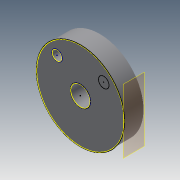
# Autodesk Inventor part: gearSupport
Saved by Autodesk Inventor 2015 (Build 190159000, 159)
## iProperties
Created: 2014-08-31
Part Number: gearSupport
Material: Generic
Document SubType Name: Modeling
Designer: shohei
Density: 1 g/cm^3
Appearance: Default
Author: shohei
Autodesk Inventor part; units mm, degrees
ref_plane "XZ Plane" through (0, 0, 0) normal (0, 1, 0) x (-1, 0, 0)
ref_plane "XY Plane" through (0, 0, 0) normal (0, 0, 1) x (1, 0, 0)
sketch "Block1" plane through (0, 0, 0) normal (0, 0, 1) x (1, 0, 0)
  circle A0 centre (0, 0) radius 20.22
  circle A1 centre (0, 12) radius 2.72
  circle A2 centre (0, 0) radius 5.22
  circle A3 centre (0, -12) radius 2.72
sketch "Block2" plane through (0, 0, 0) normal (0, 0, 1) x (1, 0, 0)
  circle A0 centre (0, 0) radius 22.72
  circle A1 centre (-12, 12) radius 2.72
  circle A2 centre (0, 0) radius 5.22
  point P0 (-4, 4)
sketch "Sketch1" plane through (0, 0, 0) normal (0, 1, 0) x (-1, 0, 0)
  circle A0 centre (0, 0) radius 22.5
  circle A1 centre (0, 0) radius 5
  line L0 (31.5, 0) -> (-31.5, 0) projected
  line L1 (0, -31.5) -> (0, 31.5) projected
  circle A2 centre (12, 12) radius 2.5
  dimension "d0" = 45
  dimension "d1" = 10
  dimension "d18" = 5
  dimension "d19" = 12
  dimension "d20" = 12
  constraints: 3 centre point, 2 coincident
  measures "d0" diameter of A0
  measures "d1" diameter of A1
  measures "d18" diameter of A2
  measures "d19" distance from line of L1 A2.centre
  measures "d20" distance from line of L0 A2.centre
ref_plane "Work Plane1" through (22.5, 0, 0) normal (1, 0, 0) x (0, 1, 0)
extrude "Extrusion4" add sketch "Sketch1" along normal blind 10 contours L0 A1 L1 A0 | A0 L1 A1 L0 | L1 A1 L0 A0 | A0 L0 A1 L1
sketch "Sketch6" plane through (0, 0, 0) normal (0, -1, 0) x (1, 0, 0)
  circle A0 centre (0, 0) radius 5 projected
  circle A1 centre (-12, 12) radius 2.5 projected
  circle A2 centre (0, 0) radius 22.5 projected
  circle A3 centre (0, 0) radius 22.72
  circle A4 centre (-12, 12) radius 2.72
  circle A5 centre (0, 0) radius 5.22
  constraints: 3 other
sketch "Sketch7" plane through (0, 0, 0) normal (0, 1, 0) x (-1, 0, 0)
  circle A0 centre (0, 0) radius 22.72
  circle A1 centre (-12, 12) radius 2.72
  circle A2 centre (0, 0) radius 5.22
equation "\"d4\" = 0.5 * d0"
body "Solid2"
